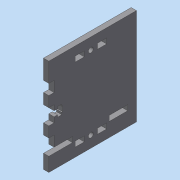
# Autodesk Inventor part: X-Anchor_Front-Side
Saved by Autodesk Inventor 2016 SP1 (Build 200210100, 210)
## iProperties
Created: 2016-03-02
Part Number: X-Anchor_Front-Side
Material: Generic
Document SubType Name: Modeling
Designer: Mohamed A.
Density: 1 g/cm^3
Appearance: Default
Author: Mohamed A.
Autodesk Inventor part; units mm, degrees
ref_plane "YZ Plane" through (0, 0, 0) normal (1, 0, 0) x (0, 1, 0)
ref_plane "XZ Plane" through (0, 0, 0) normal (0, 1, 0) x (-1, 0, 0)
ref_plane "XY Plane" through (0, 0, 0) normal (0, 0, 1) x (1, 0, 0)
sketch "Sketch2" plane through (0, 0, 0) normal (1, 0, 0) x (0, 1, 0)
  line L0 (22.5, 22.5) -> (-22.5, 22.5) construction
  line L1 (-22.5, -22.5) -> (22.5, -22.5) construction
  line L2 (22.5, -22.5) -> (22.5, 22.5) construction
  line L3 (22.5, 22.5) -> (-22.5, -22.5) construction
  line L4 (-22.5, 22.5) -> (22.5, -22.5) construction
  line L5 (-22.5, -22.5) -> (-22.5, -27.5)
  line L6 (-22.5, -27.5) -> (27.5, -27.5)
  line L7 (27.5, -27.5) -> (27.5, 27.5)
  line L8 (27.5, 27.5) -> (-22.5, 27.5)
  line L9 (-22.5, 27.5) -> (-22.5, 22.5)
  line L10 (10.5, -22.5) -> (5.25, -22.5) projected
  line L11 (10.5, -22.5) -> (10.5, -19.5) projected
  line L12 (5.25, -19.5) -> (10.5, -19.5) projected
  line L13 (5.25, -22.5) -> (5.25, -19.5) projected
  line L14 (-2.25, -22.5) -> (-7.5, -22.5) projected
  line L15 (-2.25, -22.5) -> (-2.25, -19.5) projected
  line L16 (-7.5, -19.5) -> (-2.25, -19.5) projected
  line L17 (-7.5, -22.5) -> (-7.5, -19.5) projected
  line L18 (-9, -19.5) -> (-22.5, -19.5) projected
  line L19 (-9, -19.5) -> (-9, -16.5) projected
  line L20 (-22.5, -16.5) -> (-9, -16.5) projected
  line L21 (-22.5, -19.5) -> (-22.5, -16.5) projected
  line L22 (22.5, -19.5) -> (12, -19.5) projected
  line L23 (22.5, -19.5) -> (22.5, -16.5) projected
  line L24 (12, -16.5) -> (22.5, -16.5) projected
  line L25 (12, -19.5) -> (12, -16.5) projected
  line L26 (22.5, 16.5) -> (12, 16.5) projected
  line L27 (22.5, 16.5) -> (22.5, 19.5) projected
  line L28 (12, 19.5) -> (22.5, 19.5) projected
  line L29 (12, 16.5) -> (12, 19.5) projected
  line L30 (-9, 16.5) -> (-22.5, 16.5) projected
  line L31 (-9, 16.5) -> (-9, 19.5) projected
  line L32 (-22.5, 19.5) -> (-9, 19.5) projected
  line L33 (-22.5, 16.5) -> (-22.5, 19.5) projected
  line L34 (10.5, 19.5) -> (5.25, 19.5) projected
  line L35 (10.5, 19.5) -> (10.5, 22.5) projected
  line L36 (5.25, 22.5) -> (10.5, 22.5) projected
  line L37 (5.25, 19.5) -> (5.25, 22.5) projected
  line L38 (-2.25, 19.5) -> (-7.5, 19.5) projected
  line L39 (-2.25, 19.5) -> (-2.25, 22.5) projected
  line L40 (-7.5, 22.5) -> (-2.25, 22.5) projected
  line L41 (-7.5, 19.5) -> (-7.5, 22.5) projected
  line L42 (-32.5, 0) -> (37.5, 0) construction
  line L43 (-22.5, -16.5) -> (-19.5, -16.5)
  line L44 (-19.5, -16.5) -> (-19.5, -10.5)
  line L45 (-19.5, -10.5) -> (-22.5, -10.5)
  line L46 (-22.5, 4.5) -> (-19.5, 4.5)
  line L47 (-19.5, 4.5) -> (-19.5, 1.5)
  line L48 (-19.5, 1.5) -> (-17.5, 1.5)
  line L49 (-17.5, 1.5) -> (-17.5, 2.65)
  line L50 (-17.5, 2.65) -> (-15.1, 2.65)
  line L51 (-15.1, 2.65) -> (-15.1, 1.5)
  line L52 (-15.1, 1.5) -> (-14.5, 1.5)
  line L53 (-14.5, 1.5) -> (-14.5, -1.5)
  line L54 (-14.5, -1.5) -> (-15.1, -1.5)
  line L55 (-15.1, -1.5) -> (-15.1, -2.65)
  line L56 (-15.1, -2.65) -> (-17.5, -2.65)
  line L57 (-17.5, -2.65) -> (-17.5, -1.5)
  line L58 (-19.5, -1.5) -> (-17.5, -1.5)
  line L59 (-19.5, -1.5) -> (-19.5, -4.5)
  line L60 (-19.5, -4.5) -> (-22.5, -4.5)
  line L61 (5.25, -22.5) -> (-2.25, -19.5) construction
  line L62 (5.25, -19.5) -> (-2.25, -22.5) construction
  line L63 (5.25, 19.5) -> (-2.25, 22.5) construction
  line L64 (5.25, 22.5) -> (-2.25, 19.5) construction
  circle A0 centre (1.5, 21) radius 1.4
  circle A1 centre (1.5, -21) radius 1.4
  line L65 (-22.5, 10.5) -> (-19.5, 10.5)
  line L66 (-19.5, 10.5) -> (-19.5, 16.5)
  line L67 (-22.5, 16.5) -> (-19.5, 16.5)
  line L68 (-22.5, 16.5) -> (-22.5, 10.5)
  line L69 (-22.5, 22.5) -> (-22.5, 19.5)
  line L70 (-22.5, -22.5) -> (-22.5, -16.5)
  line L71 (-22.5, -16.5) -> (-22.5, -10.5)
  line L72 (-22.5, -4.5) -> (-22.5, -10.5)
  line L73 (-22.5, 4.5) -> (-22.5, 10.5)
  line L74 (-22.5, 19.5) -> (-22.5, 16.5)
  point P0 (0, 0)
  dimension "d0" = 45
  dimension "d1" = 45
  dimension "d4" = 5
  dimension "d5" = 5
  dimension "d6" = 5
  dimension "d7" = 3
  dimension "d8" = 6
  dimension "d10" = 2
  dimension "d11" = 5
  dimension "d12" = 5.3
  dimension "d13" = 2.4
  dimension "d14" = 9
  dimension "d15" = 3
  dimension "d16" = 2.8
  dimension "d17" = 2.8
  constraints: 84 end point, 16 perpendicular, 13 point on line, 5 collinear, 4 midpoint, 3 horizontal, 3 parallel, 2 centre point, 1 vertical, 3 other
  measures "d0" distance of L1.end L1.start
  measures "d1" distance of L1.start L0.end
  measures "d4" distance of L1.start L5.end
  measures "d5" distance between parallel lines of L2 L7
  measures "d6" distance between parallel lines of L8 L0
  measures "d7" distance of L20.start L43.end
  measures "d8" distance between parallel lines of L20 L45
  measures "d10" distance between parallel lines of L59 L57
  measures "d11" distance between parallel lines of L59 L53
  measures "d12" distance between parallel lines of L50 L56
  measures "d13" distance between parallel lines of L57 L55
  measures "d14" distance between parallel lines of L46 L60
  measures "d15" distance between parallel lines of L48 L58
  measures "d16" diameter of A0
  measures "d17" diameter of A1
extrude "Extrusion1" add sketch "Sketch2" along normal blind 3 contours L70 L18 L19 L20 L44 L45 L72 L60 L59 L58 L57 L56 L55 L54 L53 L52 L51 L50 L49 L48 L47 L46 L73 L65 L66 L30 L31 L32 L69 L9 L8 L7 L6 L5 | L32 L31 L30 L33 | L26 L29 L28 L27
body "Solid1"
